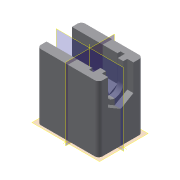
# Autodesk Inventor part: Cycl_antiBacklashY
Saved by Autodesk Inventor 2015 SP2 (Build 190223200, 223)
## iProperties
Created: 2015-04-21
Material: Genérico
Document SubType Name: Modeling
Designer: E.Beroiz
Density: 1 g/cm^3
Appearance: Valor por defecto
Description: Cycl_antiBacklashY
Author: E.Beroiz
Autodesk Inventor part; units mm, degrees
sketch "Boceto1" plane through (0, 0, 0) normal (0, 0, 1) x (1, 0, 0)
  line L0 (-16, 11.5) -> (16, 11.5)
  line L1 (16, 11.5) -> (16, -11.5)
  line L2 (16, -11.5) -> (-16, -11.5)
  line L3 (-16, -11.5) -> (-16, 11.5)
  point P0 (0, 0)
  point P1 (16, 0)
  point P2 (0, 11.5)
  dimension "d0" = 32
  dimension "d1" = 23
  constraints: 8 end point, 2 midpoint, 2 parallel, 1 horizontal, 1 horizontal alignment, 1 perpendicular, 1 vertical alignment
  measures "d0" distance of L1.end L2.end
  measures "d1" distance of L0.end L1.end
extrude "Extrusión1" add sketch "Boceto1" along normal blind 34.25
fillet "Empalme1" radius 2 4 edges at (16, -11.5, 17.125) (16, 11.5, 17.125) (-16, 11.5, 17.125) (-16, -11.5, 17.125)
sketch "Boceto2" plane through (16, -9.5, 0) normal (1, 0, 0) x (0, 0, -1)
  line L0 (-34.25, 0) -> (-34.25, 19) projected
  line L1 (-34.25, 2.918) -> (-20.45, 2.918)
  line L2 (-20.45, 2.918) -> (-16.6504, 9.5)
  line L3 (-16.6504, 9.5) -> (-20.45, 16.082)
  line L4 (-20.45, 16.082) -> (-34.25, 16.082)
  line L5 (-34.25, 2.918) -> (-34.25, 16.082)
  point P0 (0, 9.5)
  point P1 (-34.25, 9.5)
  dimension "d5" = 13.8
  dimension "d6" = 7.6
  dimension "d7" = 13.164
  constraints: 10 end point, 2 equal length, 2 point on line, 1 collinear, 1 horizontal, 1 horizontal alignment, 1 midpoint, 1 perpendicular
  measures "d5" distance of L3.end L4.end
  measures "d6" distance of L2.end L3.end
  measures "d7" distance between parallel lines of L1 L4
extrude "Extrusión2" cut sketch "Boceto2" against normal blind 3.19
sketch "Boceto3" plane through (12.81, -9.5, 0) normal (1, 0, 0) x (0, 0, -1)
  line L0 (-20.45, 2.918) -> (-34.25, 2.918) projected
  line L1 (-16.6504, 9.5) -> (-20.45, 2.918) projected
  line L2 (-20.45, 16.082) -> (-16.6504, 9.5) projected
  line L3 (-34.25, 16.082) -> (-20.45, 16.082) projected
  line L4 (-34.25, 2.918) -> (-34.25, 16.082) projected
  line L5 (-34.25, 5.0035) -> (-24.25, 5.0035)
  arc A0 (-24.25, 5.0035) -> (-24.25, 13.9965) centre (-24.25, 9.5) ccw
  line L6 (-24.25, 13.9965) -> (-34.25, 13.9965)
  line L7 (-34.25, 2.918) -> (-34.25, 16.082) projected
  line L8 (-34.25, 5.0035) -> (-34.25, 13.9965)
  point P0 (0, 9.5)
  point P1 (-34.25, 9.5)
  dimension "d10" = 10
  dimension "d11" = 8.993
  constraints: 6 end point, 2 point on circle, 2 point on line, 2 tangent, 1 centre point, 1 collinear, 1 horizontal, 1 horizontal alignment, 1 midpoint, 1 parallel
  measures "d10" distance of L6.start L6.end
  measures "d11" distance between parallel lines of L5 L6
extrude "Extrusión3" cut sketch "Boceto3" against normal blind 2.9 contours L4 L6 A0 L5
sketch "Boceto4" plane through (-16, -9.5, 0) normal (-1, 0, 0) x (0, 0, 1)
  line L0 (34.25, 16.082) -> (20.45, 16.082) projected
  line L1 (20.45, 16.082) -> (16.6504, 9.5) projected
  line L2 (16.6504, 9.5) -> (20.45, 2.918) projected
  line L3 (20.45, 2.918) -> (34.25, 2.918) projected
  line L4 (34.25, 16.082) -> (34.25, 2.918)
  line L5 (34.25, 0) -> (34.25, 2.918) projected
  point P0 (0, 9.5)
  constraints: 2 end point, 1 collinear
extrude "Extrusión4" cut sketch "Boceto4" against normal blind 23.71
sketch "Boceto5" plane through (7.71, -9.5, 0) normal (-1, 0, 0) x (0, 0, 1)
  line L0 (34.25, 17.7) -> (24.25, 17.7)
  arc A0 (24.25, 17.7) -> (24.25, 1.3) centre (24.25, 9.5) ccw
  line L1 (24.25, 1.3) -> (34.25, 1.3)
  line L2 (20.45, 2.918) -> (34.25, 2.918) projected
  line L3 (34.25, 5.0035) -> (34.25, 13.9965) projected
  line L4 (34.25, 17.7) -> (34.25, 1.3)
  line L5 (34.25, 0) -> (34.25, 2.918) projected
  point P0 (0, 9.5)
  point P1 (34.25, 9.5)
  dimension "d16" = 10
  dimension "d17" = 16.4
  constraints: 6 end point, 2 point on circle, 2 tangent, 2 vertical alignment, 1 centre point, 1 collinear, 1 horizontal, 1 horizontal alignment, 1 midpoint, 1 parallel
  measures "d16" distance of L1.end L1.start
  measures "d17" distance between parallel lines of L0 L1
extrude "Extrusión5" cut sketch "Boceto5" against normal up to surface (2.2 mm away)
sketch "Boceto6" plane through (0, 0, 0) normal (0, 0, -1) x (-1, 0, 0)
  line L0 (16, 0) -> (-7.71, 0) projected
  circle A0 centre (5, 0) radius 1.89
  circle A1 centre (-5, 0) radius 1.89
  line L1 (16, -9.5) -> (16, 9.5) projected
  point P0 (0, 0)
  dimension "d20" = 3.78
  dimension "d21" = 3.78
  dimension "d22" = 10
  dimension "d23" = 11
  constraints: 2 centre point, 2 point on line
  measures "d20" diameter of A0
  measures "d21" diameter of A1
  measures "d22" distance of A1.centre A0.centre
  measures "d23" distance from line of L1 A0.centre
extrude "Extrusión6" cut sketch "Boceto6" against normal blind 7.21
sketch "Boceto7" plane through (-5, 0, 7.21) normal (0, 0, -1) x (-1, 0, 0)
  circle A0 centre (0, 0) radius 1.89 projected
  circle A1 centre (-10, 0) radius 1.89 projected
  line L0 (3.245, -1.8735) -> (0, -3.747)
  line L1 (0, -3.747) -> (-3.245, -1.8735)
  line L2 (-3.245, -1.8735) -> (-3.245, 1.8735)
  line L3 (-3.245, 1.8735) -> (0, 3.747)
  line L4 (0, 3.747) -> (3.245, 1.8735)
  line L5 (3.245, 1.8735) -> (3.245, -1.8735)
  line L6 (-6.755, -1.8735) -> (-10, -3.747)
  line L7 (-10, -3.747) -> (-13.245, -1.8735)
  line L8 (-13.245, -1.8735) -> (-13.245, 1.8735)
  line L9 (-13.245, 1.8735) -> (-10, 3.747)
  line L10 (-10, 3.747) -> (-6.755, 1.8735)
  line L11 (-6.755, 1.8735) -> (-6.755, -1.8735)
  point P0 (-5, 0)
  dimension "d26" = 3.747
  dimension "d27" = 3.747
  constraints: 24 end point, 2 coincident, 2 vertical, 26 other
  measures "d26" distance of L4.end L0.start
  measures "d27" distance of L10.end L6.start
extrude "Extrusión7" cut sketch "Boceto7" against normal through all contours A0 | A1 | L0 L1 L2 L3 L4 L5 | L6 L7 L8 L9 L10 L11
ref_plane "Plano de trabajo1" through (0, -9.5, 0) normal (-1, 0, 0) x (0, 0, 1)
